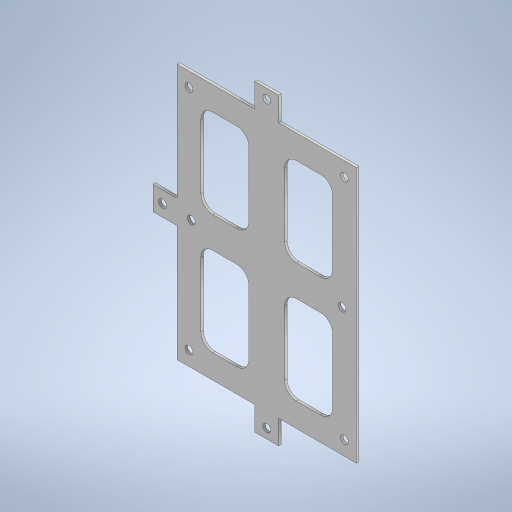
# Autodesk Inventor part: right
Saved by Autodesk Inventor 2023 (Build 270158000, 158)
## iProperties
Created: 2023-05-25
Part Number: right
Material: 一般
Document SubType Name: Sheet Metal
Designer: 310611102
Density: 1 g/cm^3
Sheet Metal Rule: Default_mm
Appearance: 預設
Author: 310611102
Autodesk Inventor part; units mm, degrees
ref_plane "YZ Plane" through (0, 0, 0) normal (1, 0, 0) x (0, 1, 0)
ref_plane "XZ Plane" through (0, 0, 0) normal (0, 1, 0) x (-1, 0, 0)
ref_plane "XY Plane" through (0, 0, 0) normal (0, 0, 1) x (1, 0, 0)
sketch "Sketch1" plane through (0, 0, 0) normal (0, 0, 1) x (1, 0, 0)
  line L0 (-37.5, 53.5) -> (37.5, 53.5)
  line L1 (37.5, 53.5) -> (37.5, -53.5)
  line L2 (37.5, -53.5) -> (-37.5, -53.5)
  line L3 (-37.5, -53.5) -> (-37.5, 53.5)
  line L4 (-37.5, 53.5) -> (37.5, -53.5) construction
  line L5 (37.5, 53.5) -> (-37.5, -53.5) construction
  line L6 (-22.5, 43.5) -> (-12.5, 43.5)
  line L7 (-7.5, 38.5) -> (-7.5, 11.5)
  line L8 (-12.5, 6.5) -> (-22.5, 6.5)
  line L9 (-27.5, 11.5) -> (-27.5, 38.5)
  line L10 (-27.5, 43.5) -> (-7.5, 6.5) construction
  line L11 (-7.5, 43.5) -> (-27.5, 6.5) construction
  arc A0 (-22.5, 43.5) -> (-27.5, 38.5) centre (-22.5, 38.5) ccw
  arc A1 (-7.5, 38.5) -> (-12.5, 43.5) centre (-12.5, 38.5) ccw
  arc A2 (-12.5, 6.5) -> (-7.5, 11.5) centre (-12.5, 11.5) ccw
  arc A3 (-27.5, 11.5) -> (-22.5, 6.5) centre (-22.5, 11.5) ccw
  line L12 (7.5, 11.5) -> (7.5, 38.5)
  arc A4 (22.5, 6.5) -> (27.5, 11.5) centre (22.5, 11.5) ccw
  arc A5 (12.5, 43.5) -> (7.5, 38.5) centre (12.5, 38.5) ccw
  arc A6 (27.5, 38.5) -> (22.5, 43.5) centre (22.5, 38.5) ccw
  arc A7 (7.5, 11.5) -> (12.5, 6.5) centre (12.5, 11.5) ccw
  line L13 (22.5, 6.5) -> (12.5, 6.5)
  line L14 (27.5, 38.5) -> (27.5, 11.5)
  line L15 (7.5, 43.5) -> (27.5, 6.5) construction
  line L16 (12.5, 43.5) -> (22.5, 43.5)
  line L17 (27.5, 43.5) -> (7.5, 6.5) construction
  line L18 (-27.5, -38.5) -> (-27.5, -11.5)
  arc A8 (-12.5, -43.5) -> (-7.5, -38.5) centre (-12.5, -38.5) ccw
  arc A9 (-22.5, -6.5) -> (-27.5, -11.5) centre (-22.5, -11.5) ccw
  arc A10 (-7.5, -11.5) -> (-12.5, -6.5) centre (-12.5, -11.5) ccw
  arc A11 (-27.5, -38.5) -> (-22.5, -43.5) centre (-22.5, -38.5) ccw
  line L19 (-12.5, -43.5) -> (-22.5, -43.5)
  line L20 (-7.5, -11.5) -> (-7.5, -38.5)
  line L21 (-27.5, -6.5) -> (-7.5, -43.5) construction
  line L22 (-22.5, -6.5) -> (-12.5, -6.5)
  line L23 (-7.5, -6.5) -> (-27.5, -43.5) construction
  line L24 (7.5, -38.5) -> (7.5, -11.5)
  arc A12 (22.5, -43.5) -> (27.5, -38.5) centre (22.5, -38.5) ccw
  arc A13 (12.5, -6.5) -> (7.5, -11.5) centre (12.5, -11.5) ccw
  arc A14 (27.5, -11.5) -> (22.5, -6.5) centre (22.5, -11.5) ccw
  arc A15 (7.5, -38.5) -> (12.5, -43.5) centre (12.5, -38.5) ccw
  line L25 (22.5, -43.5) -> (12.5, -43.5)
  line L26 (27.5, -11.5) -> (27.5, -38.5)
  line L27 (7.5, -6.5) -> (27.5, -43.5) construction
  line L28 (12.5, -6.5) -> (22.5, -6.5)
  line L29 (27.5, -6.5) -> (7.5, -43.5) construction
  circle A16 centre (-31.5, 0) radius 1.6
  line L30 (0, 0) -> (0, 8.3009)
  circle A17 centre (31.5, 0) radius 1.6
  circle A18 centre (-32.5, 47.5) radius 1.6
  line L31 (0, 0) -> (4.4939, 0)
  circle A19 centre (32.5, 47.5) radius 1.6
  circle A20 centre (-32.5, -47.5) radius 1.6
  circle A21 centre (32.5, -47.5) radius 1.6
  point P0 (-17.5, 25)
  point P1 (17.5, 25)
  point P2 (-17.5, -25)
  point P3 (17.5, -25)
  dimension "d0" = 107
  dimension "d1" = 75
  dimension "d3" = 20
  dimension "d4" = 37
  dimension "d5" = 5
  dimension "d8" = 35
  dimension "d11" = 50
  dimension "d14" = 10
  dimension "d15" = 10
  dimension "d16" = 3.2
  dimension "d17" = 6
  dimension "d18" = 3.2
  dimension "d19" = 5
  dimension "d20" = 6
  measures "d0" distance of L0.end L1.end
  measures "d1" distance of L0.start L0.end
  measures "d3" distance of L10.start L11.start
  measures "d4" distance of L11.end L10.start
  measures "d5" radius of A0
  measures "d8" distance of L9.start L12.start
  measures "d11" distance of L9.start L18.start
  measures "d14" distance between parallel lines of L0 L6
  measures "d15" distance between parallel lines of L3 L9
  measures "d16" diameter of A16
  measures "d17" distance from line of L3 A16.centre
  measures "d18" diameter of A18
  measures "d19" distance from line of L3 A18.centre
  measures "d20" distance from line of L0 A18.centre
sketch "Sketch2" plane through (0, 0, 1) normal (0, 0, 1) x (1, 0, 0)
  line L0 (37.5, 53.5) -> (37.5, -53.5)
  line L1 (-37.5, -53.5) -> (-37.5, 53.5)
  line L2 (-47.5, 5) -> (-37.5, 5)
  line L3 (-37.5, 5) -> (-37.5, -5)
  line L4 (-37.5, -5) -> (-47.5, -5)
  line L5 (-47.5, -5) -> (-47.5, 5)
  line L6 (-47.5, 5) -> (-37.5, -5) construction
  line L7 (-37.5, 5) -> (-47.5, -5) construction
  line L8 (-37.5, 53.5) -> (37.5, 53.5)
  line L9 (-5, 63.5) -> (5, 63.5)
  line L10 (5, 63.5) -> (5, 53.5)
  line L11 (5, 53.5) -> (-5, 53.5)
  line L12 (-5, 53.5) -> (-5, 63.5)
  line L13 (-5, 63.5) -> (5, 53.5) construction
  line L14 (5, 63.5) -> (-5, 53.5) construction
  line L15 (0, 0) -> (10.0151, 0)
  line L16 (-5, -63.5) -> (5, -63.5)
  line L17 (5, -63.5) -> (5, -53.5)
  line L18 (5, -53.5) -> (-5, -53.5)
  line L19 (-5, -53.5) -> (-5, -63.5)
  line L20 (-5, -63.5) -> (5, -53.5) construction
  line L21 (5, -63.5) -> (-5, -53.5) construction
  circle A0 centre (0, 59.5) radius 1.6
  circle A1 centre (-43.5, 0) radius 1.6
  circle A2 centre (0, -59.5) radius 1.6
  point P0 (-42.5, 0)
  point P1 (0, 58.5)
  point P2 (0, -58.5)
  point P3 (37.5, 38.5)
  dimension "d23" = 10
  dimension "d24" = 10
  dimension "d27" = 10
  dimension "d28" = 10
  dimension "d43" = 3.2
  dimension "d44" = 3.2
  dimension "d45" = 4
  dimension "d46" = 4
  measures "d23" distance of L9.start L9.end
  measures "d24" distance of L9.end L10.end
  measures "d27" distance of L2.start L2.end
  measures "d28" distance of L4.end L2.start
  measures "d43" diameter of A0
  measures "d44" diameter of A1
  measures "d45" distance from line of L5 A1.centre
  measures "d46" distance from line of L9 A0.centre
extrude "Plate1" add sketch "Sketch1" along normal blind 1
sheet face with bend "Face2" sketch "Sketch2" thickness 1 toward (0, 0, -1) bend radius 1 relief straight relief width 1 relief depth 0.5
bend "Bend1"
equation "\"d2\" = 厚度"
equation "\"d37\" = 折彎半徑"
equation "\"d38\" = 折彎離隙寬度"
equation "\"d40\" = 最小剩餘"
equation "\"d39\" = 折彎離隙深度"
equation "\"d41\" = 轉移半徑"
equation "\"折彎半徑\" = 厚度"
equation "\"折彎離隙寬度\" = 厚度"
equation "\"折彎離隙深度\" = 0.5 * 厚度"
equation "\"轉角離隙大小\" = 4 * 厚度"
equation "\"最小剩餘\" = 2 * 厚度"
equation "\"轉移半徑\" = 折彎半徑"
equation "\"Jacobi半徑大小\" = 折彎半徑"
equation "\"間隙大小\" = 厚度"
equation "\"厚度\" = 1"
body "Solid1"
